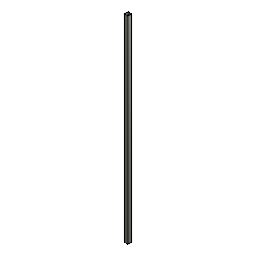
24part (Autodesk Fusion 360 design; units mm, degrees)
Autodesk Fusion 360 part; units mm, degrees
sketch "Sketch1" plane through (0, 0, 0) normal (0, 1, 0) x (1, 0, 0)
  line L0 (10, 10) -> (-10, 10)
  line L1 (-10, 10) -> (-10, -10)
  line L2 (-10, -10) -> (10, -10)
  line L3 (10, -10) -> (10, 10)
  line L4 (-8.5, 8.5) -> (-8.5, -8.5)
  line L5 (-8.5, -8.5) -> (8.5, -8.5)
  line L6 (8.5, -8.5) -> (8.5, 8.5)
  line L7 (8.5, 8.5) -> (-8.5, 8.5)
  dimension "d1" = 20
  dimension "d2" = 20
  dimension "d3" = -1.5
  constraint horizontal L0
  constraint vertical L1
  constraint horizontal L2
  constraint vertical L3
  constraint collinear L0.start L1.end origin
  constraint collinear L0.end L2.end origin
  measures "d1" distance of L0.start L0.end
  measures "d2" distance of L0.start L2.end
extrude "Extrude1" add sketch "Sketch1" along normal blind 1000
